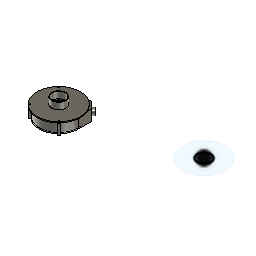
Blower V1 (Autodesk Fusion 360 design; units mm, degrees)
Autodesk Fusion 360 part; units mm, degrees
sketch "Sketch1" plane through (0, 0, 0) normal (0, 0, 1) x (1, 0, 0)
  circle A0 centre (0, 0) radius 60
  dimension "d1" = 120
  constraint coincident A0.centre origin
  measures "d1" diameter of A0
extrude "Extrude1" add sketch "Sketch1" along normal blind 3 makes body 1
sketch "Sketch2" plane through (0, 0, 3) normal (0, 0, 1) x (-1, 0, 0)
  circle A0 centre (0, 0) radius 60
  circle A1 centre (0, 0) radius 59
  circle A2 centre (0, 0) radius 60
  dimension "d4" = 118
  constraint coincident A0.centre A1.centre
  constraint concentric A1 A2
  measures "d4" diameter of A1
extrude "Extrude2" add sketch "Sketch2" along normal blind 30 bodies 1
sketch "Sketch3" plane through (0, 0, 3) normal (0, 0, 1) x (-1, 0, 0)
  circle A0 centre (0, 0) radius 59
  circle A1 centre (0, 0) radius 16.5
  dimension "d7" = 33
  constraint coincident A0.centre A1.centre
  measures "d7" diameter of A1
extrude "Extrude3" add sketch "Sketch3" against normal blind 28 contours A1 bodies 1
sketch "Sketch4" plane through (0, 0, 3) normal (0, 0, 1) x (-1, 0, 0)
  circle A0 centre (0, 0) radius 59
  circle A1 centre (0, 0) radius 15
  dimension "d10" = 30
  constraint coincident A0.centre A1.centre
  measures "d10" diameter of A1
extrude "Extrude4" cut sketch "Sketch4" against normal blind 25 contours A1 bodies 1
sketch "Sketch5" plane through (0, 0, -22) normal (0, 0, 1) x (-1, 0, 0)
  circle A0 centre (0, 0) radius 15
  circle A1 centre (0, 0) radius 4
  dimension "d13" = 8
  constraint coincident A0.centre A1.centre
  measures "d13" diameter of A1
extrude "Extrude5" cut sketch "Sketch5" against normal blind 3 contours A1 bodies 1
sketch "Sketch6" plane through (0, 0, 0) normal (0, 0, 1) x (1, 0, 0)
  circle A0 centre (0, 8) radius 1.5
  circle A1 centre (0, -7) radius 1.5
  circle A2 centre (-9, 0) radius 1.5
  circle A3 centre (9, 0) radius 1.5
  dimension "d16" = 3
  dimension "d17" = 3
  dimension "d18" = 9
  dimension "d19" = 9
  dimension "d20" = 3
  dimension "d21" = 3
  measures "d16" diameter of A0
  measures "d17" diameter of A1
  measures "d18" distance of origin A2.centre
  measures "d19" distance of origin A3.centre
  measures "d20" diameter of A2
  measures "d21" diameter of A3
extrude "Extrude6" cut sketch "Sketch6" against normal blind 30 bodies 1
sketch "Sketch7" plane through (0, 0, 0) normal (1, 0, 0) x (0, 1, 0)
  line L0 (10, -15) -> (-12.6939, -15)
  line L1 (-12.6939, -15) -> (-12.6939, -20.7765)
  line L2 (-12.6939, -20.7765) -> (10, -20.7765)
  line L3 (10, -20.7765) -> (10, -15)
  constraint horizontal L0
  constraint vertical L1
  constraint horizontal L2
  constraint vertical L3
extrude "Extrude7" cut sketch "Sketch7" along normal blind 30 bodies 1
sketch "Sketch8" plane through (0, 0, 3) normal (0, 0, 1) x (-1, 0, 0)
  circle A0 centre (0, 0) radius 15
  circle A1 centre (0, 0) radius 59
  line L0 (-60, 0, 30) -> (-60, -60, 30)
  line L1 (-60, -60, 30) -> (0, -60, 30)
  arc A2 through (-60, 0, 30) (-42.4264, -42.4264, 30) (0, -60, 30)
extrude "Extrude8" add sketch "Sketch8" against normal blind 33 contours L0 L1 A2 in plane through (0, 0, 33) normal (0, 0, 1) bodies 1
sketch "Sketch9" plane through (0, 0, 33) normal (0, 0, 1) x (-1, 0, 0)
  circle A0 centre (0, 0) radius 59
  arc A1 (0, -60) -> (-60, 0) centre (0, 0) ccw
  line L0 (-60, 0) -> (-60, -60)
  line L1 (-60, -60) -> (0, -60)
  line L2 (-60, -60) -> (-40, -60)
  line L3 (-60, -60) -> (-60, -40)
  line L4 (-40, -60) -> (-60, -40)
  constraint coincident L0.end L1.start
  constraint coincident L1 L2.end
  constraint perpendicular L0 L2
  constraint coincident L0 L3.end
  constraint perpendicular L2 L3
extrude "Extrude9" cut sketch "Sketch9" against normal blind 33 contours L0 L1 L2 L3 L4 bodies 1
sketch "Sketch10" plane through (50, 50, 0) normal (0.707107, 0.707107, 0) x (-0.707107, 0.707107, 0)
  line L0 (14.1421, 33) -> (-14.1421, 33)
  line L1 (-14.1421, 33) -> (-14.1421, 0)
  line L2 (-14.1421, 0) -> (14.1421, 0)
  line L3 (14.1421, 0) -> (14.1421, 33)
  circle A0 centre (0, 16.5) radius 7.5
  circle A1 centre (0, 16.5) radius 9.5
  dimension "d30" = 15
  dimension "d31" = 19
  constraint concentric A0 A1
  measures "d30" diameter of A0
  measures "d31" diameter of A1
extrude "Extrude10" add sketch "Sketch10" along normal blind 8 contours A1 bodies 1
hole "Hole1" at (50, 50, 16.5) direction (-0.707107, -0.707107, 0) diameter 15 depth 20 tip angle 180 bodies 1
sketch "Sketch11" plane through (0, 0, 3) normal (0, 0, 1) x (-1, 0, 0)
  circle A0 centre (0, 0) radius 15
  circle A1 centre (0, 0) radius 59
  line L0 (-38.655, -58.5908) -> (-58.655, -38.5908)
  line L1 (-58.655, -38.5908) -> (-48.655, -48.5908)
  line L2 (-48.655, -48.5908) -> (-42.291, -54.9547)
  line L3 (-48.655, -48.5908) -> (-55.0189, -42.2268)
  line L4 (-55.0189, -42.2268) -> (-55.0189, -9.4263)
  line L5 (-42.291, -54.9547) -> (2.8795, -54.9547)
  line L6 (2.8795, -54.9547) -> (-55.0189, -9.4263)
  dimension "d37" = 9
  dimension "d38" = 9
  constraint midpoint L0 L1.end
  constraint parallel L0 L1
  constraint parallel L0 L2
  constraint parallel L1 L3
  constraint vertical L4
  constraint horizontal L5
  measures "d37" distance of L1.end L2.end
  measures "d38" distance of L1.end L3.end
extrude "Extrude11" cut sketch "Sketch11" along normal blind 25 contours A1 L0 L1 L2 L3 L4 L5 bodies 1
sketch "Sketch12" plane through (0, 0, 0) normal (0, 0, 1) x (1, 0, 0)
  line L0 (0, 0) -> (-0.0063, 0.0063)
  line L1 (0, 0) -> (59.9985, 0) construction
  line L2 (0, 0) -> (-44.5477, 44.5477)
  circle A0 centre (-44.5477, 44.5477) radius 2.1
  line L3 (-44.5477, 44.5477) -> (-41.7193, 41.7193)
  line L4 (-41.7193, 41.7193) -> (-43.8406, 39.598)
  line L5 (-41.7193, 41.7193) -> (-39.598, 43.8406)
  line L6 (-43.8406, 39.598) -> (-49.1439, 44.9013)
  line L7 (-39.598, 43.8406) -> (-44.9013, 49.1439)
  line L8 (-39.598, 43.8406) -> (-31.598, 43.8406) construction
  line L9 (-44.9013, 49.1439) -> (-49.1439, 44.9013)
  line L10 (0, 0) -> (44.5477, -44.5477)
  line L11 (0, 0) -> (63, 0) construction
  circle A1 centre (44.5477, -44.5477) radius 2.1
  line L12 (44.5477, -44.5477) -> (41.7193, -41.7193)
  line L13 (41.7193, -41.7193) -> (43.8406, -39.598)
  line L14 (41.7193, -41.7193) -> (39.598, -43.8406)
  line L15 (39.598, -43.8406) -> (44.9013, -49.1439)
  line L16 (43.8406, -39.598) -> (49.1439, -44.9013)
  line L17 (49.1439, -44.9013) -> (44.9013, -49.1439)
  line L18 (-0.0063, 0.0063) -> (-44.554, -44.5414)
  circle A2 centre (-44.554, -44.5414) radius 2.1
  line L19 (-44.554, -44.5414) -> (-41.7256, -41.713)
  line L20 (-41.7256, -41.713) -> (-39.6043, -43.8343)
  line L21 (-41.7256, -41.713) -> (-43.8469, -39.5917)
  line L22 (-39.6043, -43.8343) -> (-44.9076, -49.1376)
  line L23 (-39.6043, -43.8343) -> (-31.8208, -43.8343) construction
  line L24 (-43.8469, -39.5917) -> (-49.1502, -44.895)
  line L25 (-43.8469, -39.5917) -> (-36.0635, -39.5917) construction
  line L26 (-44.9076, -49.1376) -> (-49.1502, -44.895)
  dimension "d92" = 63
  dimension "d93" = 4.2
  dimension "d94" = 4
  dimension "d95" = 3
  dimension "d96" = 3
  dimension "d97" = 7.5
  dimension "d98" = 135
  dimension "d99" = 7.5
  dimension "d101" = 45
  dimension "d102" = 63
  dimension "d103" = 4.2
  dimension "d104" = 4
  dimension "d105" = 3
  dimension "d106" = 3
  dimension "d107" = 90
  dimension "d108" = 7.5
  dimension "d109" = 7.5
  dimension "d110" = 63
  dimension "d111" = 4.2
  dimension "d112" = 4
  dimension "d113" = 3
  dimension "d114" = 3
  dimension "d115" = 135
  dimension "d116" = 7.5
  dimension "d117" = 135
  dimension "d118" = 7.5
  constraint horizontal L1
  constraint coincident L0.start L1.start
  constraint parallel L0 L2
  constraint coincident L2.end A0.centre
  constraint parallel L2 L3
  constraint perpendicular L3 L4
  constraint perpendicular L2 L5
  constraint perpendicular L4 L6
  constraint horizontal L8
  constraint perpendicular L5 L7
  constraint horizontal L11
  constraint coincident L10.end A1.centre
  constraint parallel L10 L12
  constraint perpendicular L10 L13
  constraint perpendicular L10 L14
  constraint perpendicular L13 L16
  constraint perpendicular L2 L18
  constraint coincident L18.end A2.centre
  constraint parallel L18 L19
  constraint perpendicular L19 L20
  constraint perpendicular L19 L21
  constraint horizontal L23
  constraint horizontal L25
  measures "d92" distance of L0.start L2.end
  measures "d93" diameter of A0
  measures "d94" distance of L2.end L3.end
  measures "d95" distance of L3.end L4.end
  measures "d96" distance of L3.end L5.end
  measures "d97" distance of L4.end L6.end
  measures "d98" angle of L7 L8
  measures "d99" distance of L5.end L7.end
  measures "d101" angle of L10 L11
  measures "d102" distance of L0.start L10.end
  measures "d103" diameter of A1
  measures "d104" distance of L10.end L12.end
  measures "d105" distance of L12.end L13.end
  measures "d106" distance of L12.end L14.end
  measures "d107" angle of L14 L15
  measures "d108" distance of L14.end L15.end
  measures "d109" distance of L13.end L16.end
  measures "d110" distance of L0.end L18.end
  measures "d111" diameter of A2
  measures "d112" distance of L18.end L19.end
  measures "d113" distance of L19.end L20.end
  measures "d114" distance of L19.end L21.end
  measures "d115" angle of L22 L23
  measures "d116" distance of L20.end L22.end
  measures "d117" angle of L24 L25
  measures "d118" distance of L21.end L24.end
extrude "Extrude12" add sketch "Sketch12" along normal blind 33 bodies 1
sketch "Sketch13" plane through (0, 0, 0) normal (0, 0, 1) x (1, 0, 0)
  circle A0 centre (250, 125) radius 66
  line L0 (250, 125) -> (301.6066, 161.1353)
  line L1 (250, 125) -> (312.5, 125) construction
  line L2 (250, 125) -> (286.1353, 73.3934)
  line L3 (250, 125) -> (213.8647, 176.6066)
  circle A1 centre (286.1353, 73.3934) radius 2.1
  circle A2 centre (301.6066, 161.1353) radius 2.1
  circle A3 centre (213.8647, 176.6066) radius 2.1
  dimension "d63" = 132
  dimension "d64" = 63
  dimension "d65" = 35
  dimension "d66" = 63
  dimension "d67" = 63
  dimension "d68" = 4.2
  dimension "d69" = 4.2
  dimension "d70" = 4.2
  constraint horizontal L1
  constraint coincident A0.centre L0.start
  constraint perpendicular L0 L2
  constraint perpendicular L0 L3
  constraint coincident L2.end A1.centre
  constraint coincident L0.end A2.centre
  constraint coincident L3.end A3.centre
  measures "d63" diameter of A0
  measures "d64" distance of A0.centre L0.end
  measures "d65" angle of L0 L1
  measures "d66" distance of A0.centre L2.end
  measures "d67" distance of A0.centre L3.end
  measures "d68" diameter of A1
  measures "d69" diameter of A2
  measures "d70" diameter of A3
extrude "Extrude13" add sketch "Sketch13" along normal blind 3 separate body makes body 2
sketch "Sketch14" plane through (0, 0, 3) normal (0, 0, 1) x (-1, 0, 0)
  circle A0 centre (-213.8647, -176.6066) radius 2.1
  circle A1 centre (-301.6066, -161.1353) radius 2.1
  circle A2 centre (-286.1353, -73.3934) radius 2.1
  circle A3 centre (-250, -125) radius 66
  circle A4 centre (-250, -125) radius 20
  circle A5 centre (-250, -125) radius 21.5
  dimension "d73" = 40
  dimension "d74" = 43
  constraint concentric A3 A4
  constraint concentric A4 A5
  measures "d73" diameter of A4
  measures "d74" diameter of A5
hole "Hole2" at (249.9484, 124.9639, 3) direction (0, 0, -1) diameter 40 depth 7 tip angle 180 bodies 2
extrude "Extrude14" add sketch "Sketch14" along normal blind 20 contours A5 bodies 2
copy_body "Body->Comp1" bodies 1 removing the originals makes body 3 in component "Duct"
copy_body "Body->Comp2" bodies 2 removing the originals makes body 4 in component "Top"
component "Duct" placed x (1, 0, 0) y (0, 1, 0) z (0, 0, 1) at (0, 0, 0)
component "Top" placed x (-0.984808, -0.173648, 0) y (0.173648, -0.984808, 0) z (0, 0, 1) at (224.4896, 166.5193, 33)
